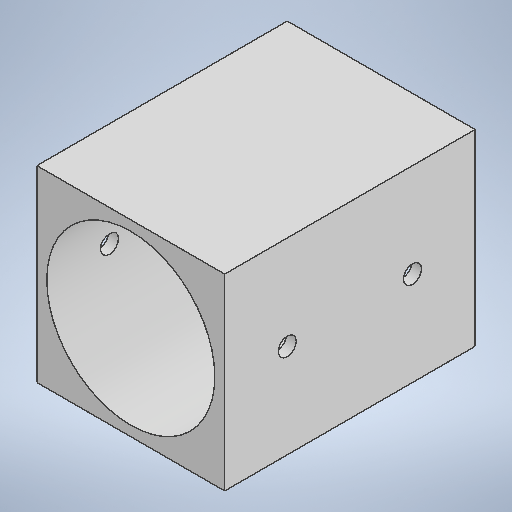
# Autodesk Inventor part: Bohrschablone_Oben
Saved by Autodesk Inventor 2026.2 (Build 302298000, 298)
## iProperties
Created: 2026-03-24
Part Number: Bohrschablone_Oben
Material: Generic
Document SubType Name: Modeling
Designer: Paco Ariel
Density: 1 g/cm^3
Appearance: Default
Author: Paco Ariel
Autodesk Inventor part; units mm, degrees
ref_plane "YZ Plane" through (0, 0, 0) normal (1, 0, 0) x (0, 1, 0)
ref_plane "XZ Plane" through (0, 0, 0) normal (0, 1, 0) x (-1, 0, 0)
ref_plane "XY Plane" through (0, 0, 0) normal (0, 0, 1) x (1, 0, 0)
sketch "Sketch1" plane through (0, 0, 0) normal (1, 0, 0) x (0, 1, 0)
  line L0 (0, 0) -> (0, -15)
  line L1 (0, -15) -> (0, -45)
  line L2 (0, -45) -> (0, -60)
  dimension "d0" = 15
  dimension "d2" = 30
  dimension "d3" = 15
  constraints: 6 end point, 2 coincident, 2 point on line, 1 vertical
  measures "d0" distance of L0.start L0.end
  measures "d2" distance of L0.end L1.end
  measures "d3" distance of L1.end L2.end
sketch "Sketch2" plane through (0, 0, 0) normal (0, 0, 1) x (1, 0, 0)
  line L0 (-22.5, 22.5) -> (22.5, 22.5)
  line L1 (22.5, 22.5) -> (22.5, -22.5)
  line L2 (22.5, -22.5) -> (-22.5, -22.5)
  line L3 (-22.5, -22.5) -> (-22.5, 22.5)
  line L4 (-22.5, 22.5) -> (22.5, -22.5) construction
  line L5 (22.5, 22.5) -> (-22.5, -22.5) construction
  circle A0 centre (0, 0) radius 20.125
  dimension "d6" = 45
  dimension "d7" = 45
  dimension "d8" = 40.25
  constraints: 12 end point, 2 midpoint, 2 parallel, 1 centre point, 1 coincident, 1 horizontal, 1 perpendicular
  measures "d6" distance of L1.end L2.end
  measures "d7" distance of L0.end L1.end
  measures "d8" diameter of A0
extrude "Extrusion1" add sketch "Sketch2" against normal blind 60
hole "Hole1" at (0, 0, -15) at (0, 0, -45) direction (-1, 0, 0) diameter 4.3 end through all both
body "Solid1"
